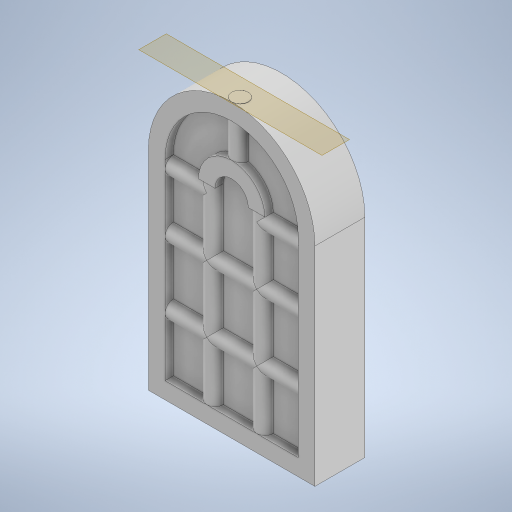
# Autodesk Inventor part: WindowofShip11
Saved by Autodesk Inventor 2023 (Build 270158000, 158)
## iProperties
Created: 2023-10-26
Part Number: WindowofShip11
Material: Generic
Document SubType Name: Modeling
Designer: student
Density: 1 g/cm^3
Appearance: Default
Author: student
Autodesk Inventor part; units mm, degrees
ref_plane "YZ Plane" through (0, 0, 0) normal (1, 0, 0) x (0, 1, 0)
ref_plane "XY Plane" through (0, 0, 0) normal (0, 0, 1) x (1, 0, 0)
sketch "Sketch1" plane through (0, 0, 0) normal (0, 0, 1) x (1, 0, 0)
  line L0 (0, 0) -> (1000, 0)
  line L1 (1000, 0) -> (1000, 1250)
  line L2 (1000, 1250) -> (0, 1250)
  line L3 (0, 1250) -> (0, 0)
  dimension "d0" = 1000
  dimension "d1" = 1250
  constraints: 8 end point, 2 parallel, 1 horizontal, 1 perpendicular
  measures "d0" distance of L1.end L2.end
  measures "d1" distance of L0.end L1.end
extrude "Extrusion1" add sketch "Sketch1" along normal blind 100
sketch "Sketch2" plane through (0, 0, 0) normal (0, 0, -1) x (-1, 0, 0)
  line L0 (-1000, 1250) -> (0, 1250) projected
  circle A0 centre (-500, 1250) radius 500
  point P0 (0, 0)
  dimension "d4" = 1000
  constraints: 1 centre point, 1 midpoint
  measures "d4" diameter of A0
extrude "Extrusion2" add sketch "Sketch2" against normal blind 100 contours A0 L0 picked at (-386.6625, 1415.594)
sketch "Sketch3" plane through (0, 0, 0) normal (0, -1, 0) x (1, 0, 0)
  line L0 (0, 100) -> (1000, 100) projected
  circle A0 centre (350, 100) radius 50
  circle A1 centre (650, 100) radius 50
  line L1 (0, 0) -> (0, 100) projected
  line L2 (1000, 0) -> (1000, 100) projected
  point P0 (1000, 50)
  dimension "d7" = 100
  dimension "d8" = 100
  dimension "d9" = 350
  dimension "d10" = 350
  constraints: 2 centre point, 2 point on line, 1 midpoint
  measures "d7" diameter of A0
  measures "d8" diameter of A1
  measures "d9" distance from line of A0.centre L1
  measures "d10" horizontal distance of point (1000, 50) A1.centre
extrude "Extrusion3" add sketch "Sketch3" against normal blind 1250
sketch "Sketch4" plane through (1000, 0, 100) normal (1, 0, 0) x (0, 0, -1)
  line L0 (0, 1250) -> (0, 0) projected
  circle A0 centre (0, 450) radius 50
  circle A1 centre (0, 850) radius 50
  line L1 (100, 0) -> (0, 0) projected
  line L2 (100, 1250) -> (0, 1250) projected
  dimension "d13" = 100
  dimension "d14" = 100
  dimension "d15" = 450
  dimension "d16" = 400
  dimension "d17" = 400
  constraints: 2 centre point, 1 point on line
  measures "d13" diameter of A0
  measures "d14" diameter of A1
  measures "d15" distance from line of A0.centre L1
  measures "d16" distance of A1.centre A0.centre
  measures "d17" distance from line of L2 A1.centre
extrude "Extrusion4" add sketch "Sketch4" against normal blind 1000
sketch "Sketch5" plane through (0, 0, 100) normal (0, 0, 1) x (1, 0, 0)
  line L0 (700, 1250) -> (600, 1250) projected
  line L1 (400, 1250) -> (300, 1250) projected
  arc A0 (600, 1250) -> (400, 1250) centre (500, 1250) ccw
  arc A1 (700, 1250) -> (300.0458, 1245.6914) centre (500.0458, 1245.7187) ccw
  point P0 (0, 0)
  point P1 (300.0917, 1250)
  dimension "d20" = 100
  dimension "d21" = 200
  constraints: 4 point on circle, 2 centre point
  measures "d20" radius of A0
  measures "d21" radius of A1
extrude "Extrusion5" add sketch "Sketch5" along normal blind 50
sketch "Sketch6" plane through (1000, 0, 100) normal (1, 0, 0) x (0, 0, -1)
  line L0 (0, 900) -> (0, 1250) projected
  circle A0 centre (0, 1200) radius 50
  line L1 (100, 1250) -> (0, 1250) projected
  point P0 (100, 0)
  dimension "d24" = 100
  dimension "d25" = 50
  constraints: 1 centre point, 1 point on line
  measures "d24" diameter of A0
  measures "d25" distance from line of L1 A0.centre
extrude "Extrusion6" add sketch "Sketch6" against normal up to surface
sketch "Sketch7" plane through (0, 0, 0) normal (-1, 0, 0) x (0, 0, 1)
  line L0 (100, 900) -> (100, 1250) projected
  circle A0 centre (100, 1200) radius 50
  line L1 (0, 1250) -> (100, 1250) projected
  point P0 (0, 0)
  dimension "d28" = 100
  dimension "d29" = 50
  constraints: 1 centre point, 1 point on line
  measures "d28" diameter of A0
  measures "d29" distance from line of A0.centre L1
extrude "Extrusion7" add sketch "Sketch7" against normal up to surface
ref_plane "Work Plane1" through (0, 1750, 0) normal (0, 1, 0) x (-1, 0, 0)
sketch "Sketch8" plane through (0, 1750, 0) normal (0, 1, 0) x (-1, 0, 0)
  line L0 (-400, 100) -> (-600, 100) projected
  circle A0 centre (-500, 100) radius 50
  point P0 (0, 0)
  dimension "d33" = 100
  constraints: 1 centre point, 1 midpoint
  measures "d33" diameter of A0
extrude "Extrusion8" add sketch "Sketch8" against normal up to surface
sketch "Sketch9" plane through (0, 0, 100) normal (0, 0, 1) x (1, 0, 0)
  line L0 (1000, 1150) -> (700, 1150) projected
  line L1 (900, 1150) -> (900, 902.0075)
  line L2 (1000, 900) -> (1000, 1150) projected
  line L3 (1000, 800) -> (700, 800) projected
  line L4 (900, 800) -> (900, 0)
  line L5 (0, 0) -> (1000, 0) projected
  line L6 (100, 0) -> (100, 1250)
  line L7 (0, 1250) -> (300, 1250) projected
  line L8 (0, 800) -> (0, 500) projected
  arc A0 (1000, 1250) -> (0, 1250) centre (500, 1250) ccw projected
  line L9 (0, 1250) -> (0, 0) projected
  line L10 (0, 1250) -> (0, 0)
  line L11 (700, 1250) -> (1000, 1250) projected
  line L12 (1000, 1250) -> (1000, 0)
  arc A1 (900, 1250) -> (100, 1250) centre (500, 1250) ccw
  point P0 (900, 1026.0038)
  point P1 (100, 625)
  dimension "d36" = 100
  dimension "d37" = 100
  constraints: 10 end point, 5 point on line, 3 vertical, 2 midpoint, 2 point on circle, 1 centre point, 1 collinear, 1 perpendicular, 1 tangent
  measures "d36" distance from line of point (900, 1026.004) L2
  measures "d37" distance from line of point (100, 625) L8
extrude "Extrusion9" add sketch "Sketch9" along normal blind 50 contours L11 A1 L7 A0
sketch "Sketch10" plane through (0, 0, 100) normal (0, 0, 1) x (1, 0, 0)
  arc A0 (900, 1250) -> (550, 1646.8627) centre (500, 1250) ccw projected
  line L0 (900, 1250) -> (900, 0)
  line L1 (1000, 0) -> (1000, 1250) projected
  line L2 (1000, 1250) -> (1000, 0)
  line L3 (1000, 1150) -> (700, 1150) projected
  line L4 (900, 1150) -> (1000, 1150)
  line L5 (0, 0) -> (1000, 0) projected
  line L6 (900, 0) -> (1000, 0)
  constraints: 8 end point, 2 collinear, 2 point on line, 1 horizontal, 1 vertical
extrude "Extrusion10" add sketch "Sketch10" along normal blind 50
sketch "Sketch11" plane through (0, 0, 100) normal (0, 0, 1) x (1, 0, 0)
  line L0 (100, 1250) -> (100, 0)
  line L1 (0, 0) -> (300, 0) projected
  line L2 (0, 0) -> (0, 1250)
  line L3 (0, 400) -> (0, 0) projected
  line L4 (0, 1250) -> (100, 1250)
  line L5 (0, 0) -> (100, 0)
  constraints: 8 end point, 2 collinear, 1 perpendicular, 1 point on line, 1 vertical
extrude "Extrusion11" add sketch "Sketch11" along normal blind 50
sketch "Sketch12" plane through (0, 0, 100) normal (0, 0, 1) x (1, 0, 0)
  line L0 (700, 1250) -> (900, 1250) projected
  line L1 (900, 1250) -> (900, 1150)
  line L2 (900, 1150) -> (1000, 1150)
  line L3 (900, 1250) -> (1000, 1250) projected
  line L4 (1000, 1150) -> (1000, 1250)
  line L5 (1000, 1250) -> (900, 1250)
  point P0 (0, 0)
  constraints: 8 end point, 3 perpendicular
extrude "Extrusion12" add sketch "Sketch12" along normal blind 50
sketch "Sketch13" plane through (0, 0, 100) normal (0, 0, 1) x (1, 0, 0)
  line L0 (0, 1250) -> (0, 0) projected
  line L1 (0, 100) -> (1042, 100)
  line L2 (400, 0) -> (600, 0) projected
  line L3 (0, 0) -> (100, 0) projected
  line L4 (0, 100) -> (0, 0)
  line L5 (900, 0) -> (1000, 0) projected
  line L6 (0, 0) -> (1000, 0)
  line L7 (1000, 0) -> (1000, 100)
  line L8 (1000, 0) -> (1000, 1250) projected
  point P0 (500, 0)
  point P1 (521, 100)
  dimension "d46" = 100
  constraints: 8 end point, 3 point on line, 2 midpoint, 1 collinear, 1 horizontal, 1 vertical
  measures "d46" vertical distance of point (500, 0) point (521, 100)
extrude "Extrusion13" add sketch "Sketch13" along normal blind 50
sketch "Sketch14" plane through (0, 0, 0) normal (0, 0, -1) x (-1, 0, 0)
  arc A0 (-500, 1750) -> (-1000, 1250) centre (-500, 1250) ccw projected
  line L0 (-1000, 0) -> (-1000, 1250) projected
  line L1 (-1000, 1250) -> (-1000, 0)
  line L2 (0, 0) -> (-1000, 0) projected
  line L3 (-1000, 0) -> (0, 0)
  arc A1 (0, 1250) -> (-500, 1750) centre (-500, 1250) ccw projected
  line L4 (0, 0) -> (0, 1250)
  line L5 (0, 1250) -> (-1000, 1250)
  circle A2 centre (-500, 1250) radius 500
  constraints: 8 end point, 2 collinear, 2 perpendicular, 1 centre point, 1 coincident, 1 tangent
extrude "Extrusion14" add sketch "Sketch14" along normal blind 150
body "Solid1"
